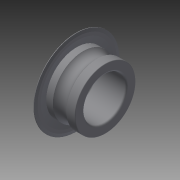
# Autodesk Inventor part: 6202-Z_PART1
Saved by Autodesk Inventor 2014 SP2 (Build 180246200, 246)
## iProperties
Created: 2019-12-08
Part Number: 6202-Z_PART1
Material: Generic
Catalog Web Link: www.cadenas.de
Description: -Deep groove ball bearings
Vendor: SKF
Document SubType Name: Modeling
Designer: psadmin
Manufacturer: SKF
Mass: 1.94506 g
Surface Area: 23.7309 cm^2
Volume: 1.94506 cm^3
Density: 1 g/cm^3
Appearance: PSOLRGB-175-175-175
Category: PARTsolutions
Company: SKF
Title: 6202-Z_PART1
Author: Cadenas PARTsolutions
Comments: Deep groove ball bearings
PSOL_IDENT_0: {$CADENAS_DATA\23d-libs\skf\bearings_units_and_housings\ball_bearings\deep_groove_ball_bearings\bb1_
PSOL_IDENT_1: 001_101.prj},191 {VTYP=3D},{NB=6202-Z_PART1},{LINA=6202-Z_PART1},{NN=BB1_001_101_PART1},{NOPRJ=TRUE}
PSOL_IDENT_2: ,{DATE=04.12.2019 15:23:41},{GEOMDATE=20.11.2019 09:53:42},{VERSION=},{LINEID=12130},{WBVAR=},{WBNUM
PSOL_IDENT_3: ERIC=}  {NB=6202-Z_PART1},{LINA=6202-Z_PART1},{KT=DUMMY},{PRODUCTID=1050050202},{DESIGNATION=6202-Z}
PSOL_IDENT_4: ,{DD=15.000},{D=35.000},{B=11.000},{C=0.000},{DD1=21.70},{DD2=0.00},{D1=0.00},{D2=30.50},{D3=0.000},
PSOL_IDENT_5: {D4=0.000},{HH=MIN},{BB=0.000},{FF=0.00},{R0MAX=MIN},{R0=MIN},{R12=0.60},{PITCH=25.26},{DW=6.000},{D
PSOL_IDENT_6: DAMIN=19.200},{DDAMAX=21.600},{DDBMIN=MIN},{DDBMAX=MIN},{DBMIN=MIN},{DAMAX=30.800},{BBAMIN=MIN},{CAM
PSOL_IDENT_7: AX=MIN},{RAMAX=0.600},{LOAD1=8.060},{LOAD2=3.750},{LOAD3=0.160},{SPEED1=43000},{SPEED2=28000},{KR=0.
PSOL_IDENT_8: 025},{F0=13.000},{Z=8},{II=1},{MASS=0.046},{BEARING=6202-Z},{RING=},{HELP=2.860},{HELP2=2.250},{DD1A
PSOL_IDENT_9: LG=10.850},{YALG=10.850},{PITCH1=25.260},{DW1=6.000},{YALG1=14.640},{HALG1=2.860},{SH=10.850},{CU=1.
PSOL_IDENT_10: 000},{DESIGN=dgbbz},{HALG=3.35},{B1=0},{ALGO=1.000}
NT: Deep groove ball bearings
NB: 6202-Z_PART1
NBSYN: $DESIGNATION._PART1
LINA: 6202-Z_PART1
SUPPLIER: SKF
ARTICLENO: 6202-Z_PART1
BOMINFO: 6202-Z_PART1
CREATOR: CADENAS GmbH
Autodesk Inventor part; units mm, degrees
ref_plane "YZ Plane" through (0, 0, 0) normal (1, 0, 0) x (0, 1, 0)
ref_plane "XZ Plane" through (0, 0, 0) normal (0, 1, 0) x (-1, 0, 0)
ref_plane "XY Plane" through (0, 0, 0) normal (0, 0, 1) x (1, 0, 0)
sketch "Sketch_62" plane through (0, 0, 0) normal (0, 0, 1) x (1, 0, 0)
  line L0 (50, 0) -> (-50, 0)
  line L1 (0, 10.65) -> (0, 8.1)
  arc A0 (0, 8.1) -> (0.6, 7.5) centre (0.6, 8.1) ccw
  line L2 (0.6, 7.5) -> (10.4, 7.5)
  arc A1 (10.4, 7.5) -> (11, 8.1) centre (10.4, 8.1) ccw
  line L3 (11, 8.1) -> (11, 10.65)
  arc A2 (11, 10.65) -> (10.8, 10.85) centre (10.8, 10.65) ccw
  line L4 (10.8, 10.85) -> (7.9149, 10.85)
  arc A3 (3.0851, 10.85) -> (7.9149, 10.85) centre (5.5, 12.63) ccw
  line L5 (3.0851, 10.85) -> (0.2, 10.85)
  arc A4 (0.2, 10.85) -> (0, 10.65) centre (0.2, 10.65) ccw
  constraints: 12 end point, 10 point on circle, 5 centre point
revolve "Revolution1" add sketch "Sketch_62" angle 360 about axis through (50, 0, 0) along (1, 0, 0)
sketch "Sketch_63" plane through (0, 0, 0) normal (0, 0, 1) x (1, 0, 0)
  line L0 (50, 0) -> (-50, 0)
  line L1 (0.54, 15.25) -> (0.63, 14.15)
  line L2 (0.63, 14.15) -> (0.54, 13.05)
  line L3 (0.54, 13.05) -> (0.54, 10.85)
  line L4 (0.54, 10.85) -> (0.72, 10.85)
  line L5 (0.72, 10.85) -> (0.9, 13.05)
  line L6 (0.9, 13.05) -> (0.9, 14.15)
  line L7 (0.9, 14.15) -> (0.72, 15.25)
  line L8 (0.72, 15.25) -> (0.54, 15.25)
  constraints: 18 end point
revolve "Revolution2" add sketch "Sketch_63" angle 360 about axis through (50, 0, 0) along (1, 0, 0)
body "Solid1"
